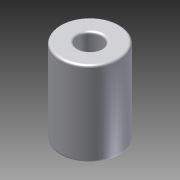
# Autodesk Inventor part: Idler
Saved by Autodesk Inventor 2012 (Build 160160000, 160)
## iProperties
Created: 2012-10-05
Part Number: Idler
Material: Default
Document SubType Name: Modeling
Designer: agmeyer
Density: 1 g/cm^3
Author: agmeyer
Autodesk Inventor part; units mm, degrees
ref_plane "YZ Plane" through (0, 0, 0) normal (1, 0, 0) x (0, 1, 0)
ref_plane "XZ Plane" through (0, 0, 0) normal (0, 1, 0) x (-1, 0, 0)
ref_plane "XY Plane" through (0, 0, 0) normal (0, 0, 1) x (1, 0, 0)
sketch "Sketch1" plane through (0, 0, 0) normal (0, 0, 1) x (1, 0, 0)
  circle A0 centre (0, 0) radius 6.35
  dimension "d0" = 12.7
  constraints: 1 centre point, 1 coincident
  measures "d0" diameter of A0
extrude "Extrusion1" add sketch "Sketch1" along normal blind 18
hole "Hole1" at (0, 0, 18) direction (0, 0, -1) diameter 5 end through all
fillet "Fillet1" radius 0.5 4 edges at (-6.35, 0, 18) (0, 2.5, 18) (0, 2.5, 0) (-6.35, 0, 0)
body "Solid1"
